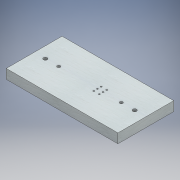
# Autodesk Inventor part: base de madera pequeña
Saved by Autodesk Inventor 2018 (Build 220112000, 112)
## iProperties
Created: 2019-05-16
Part Number: base de madera pequeña
Material: Generic
Document SubType Name: Modeling
Designer: JLVega003
Density: 1 g/cm^3
Appearance: Wood - Painted White
Author: JLVega003
Autodesk Inventor part; units mm, degrees
ref_plane "YZ Plane" through (0, 0, 0) normal (1, 0, 0) x (0, 1, 0)
ref_plane "XZ Plane" through (0, 0, 0) normal (0, 1, 0) x (-1, 0, 0)
ref_plane "XY Plane" through (0, 0, 0) normal (0, 0, 1) x (1, 0, 0)
sketch "Sketch1" plane through (0, 0, 0) normal (0, 0, 1) x (1, 0, 0)
  line L0 (-150, -75) -> (150, -75)
  line L1 (150, -75) -> (150, 75)
  line L2 (150, 75) -> (-150, 75)
  line L3 (-150, 75) -> (-150, -75)
  line L4 (-150, -75) -> (150, 75) construction
  line L5 (150, -75) -> (-150, 75) construction
  point P0 (0, 0)
  dimension "d0" = 300
  dimension "d1" = 150
  constraints: 12 end point, 2 midpoint, 2 parallel, 1 horizontal, 1 perpendicular
  measures "d0" distance of L2.end L1.end
  measures "d1" distance of L1.end L0.end
extrude "Extrusion1" add sketch "Sketch1" along normal blind 25.4
sketch "Sketch2" plane through (0, 0, 25.4) normal (0, 0, 1) x (1, 0, 0)
  line L0 (-120, 0) -> (120, 0)
  line L1 (-150, 75) -> (-150, -75) projected
  point P0 (0, 0)
  point P1 (0, 0)
  dimension "d4" = 30
  constraints: 3 coincident, 2 end point, 1 horizontal, 1 midpoint
  measures "d4" distance from line of L0.start L1
hole "Hole1" at (-120, 0, 25.4) at (120, 0, 25.4) direction (0, 0, -1) diameter 10 end through all
sketch "Sketch3" plane through (0, 0, 25.4) normal (0, 0, 1) x (1, 0, 0)
  line L0 (-84.0889, 0) -> (84.0889, 0)
  point P0 (0, 0)
  point P1 (0, 0)
  constraints: 3 coincident, 2 end point, 1 horizontal, 1 midpoint
hole "Hole2" at (-84.0889, 0, 25.4) at (84.0889, 0, 25.4) direction (0, 0, -1) diameter 8 end through all
sketch "Sketch5" plane through (0, 0, 25.4) normal (0, 0, 1) x (1, 0, 0)
  line L0 (0, 0) -> (150, 0)
  line L1 (150, -75) -> (150, 75) projected
  circle A0 centre (20, 0) radius 2
  circle A1 centre (35, 0) radius 2
  dimension "d26" = 4
  dimension "d27" = 20
  dimension "d28" = 35
  constraints: 2 centre point, 2 end point, 2 point on line, 1 equal radius, 1 midpoint
  measures "d26" diameter of A1
  measures "d27" distance of A0.centre L0.start
  measures "d28" distance of A1.centre L0.start
extrude "Extrusion2" cut sketch "Sketch5" against normal through all
pattern_linear "Rectangular Pattern1" count 2 spacing 10 along (0, -1, 0) count 2 spacing -10 along (0, -1, 0) of "Extrusion2" second direction both ways yes
body "Solid1"
